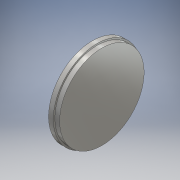
# Autodesk Inventor part: snow_can_top
Saved by Autodesk Inventor 2016 (Build 200138000, 138)
## iProperties
Created: 2017-01-14
Part Number: snow_can_top
Material: Generic
Document SubType Name: Modeling
Designer: hesaon
Density: 1 g/cm^3
Appearance: Default
Author: hesaon
Autodesk Inventor part; units mm, degrees
ref_plane "YZ Plane" through (0, 0, 0) normal (1, 0, 0) x (0, 1, 0)
ref_plane "XZ Plane" through (0, 0, 0) normal (0, 1, 0) x (-1, 0, 0)
ref_plane "XY Plane" through (0, 0, 0) normal (0, 0, 1) x (1, 0, 0)
sketch "Sketch1" plane through (0, 0, 0) normal (0, 1, 0) x (-1, 0, 0)
  line L0 (0, 27.75) -> (3, 27.75)
  line L1 (3, 27.75) -> (3, 25.75)
  line L2 (-3, 25.75) -> (-3, 23.75)
  line L3 (8, 13.5) -> (8, 0)
  line L4 (-3, 26.75) -> (-3, 0)
  line L5 (8, 0) -> (0, 0)
  arc A0 (8, 13.5) -> (0, 23.75) centre (-2.5664, 13.5) ccw
  arc A1 (0, 25.75) -> (0, 23.75) centre (0, 24.75) ccw
  line L6 (0, 26.75) -> (-3, 26.75)
  line L7 (-3, 26.75) -> (-3, 25.75)
  line L8 (3, 25.75) -> (0, 25.75)
  line L9 (0, 27.75) -> (0, 26.75)
  line L10 (0, 0) -> (-3, 0)
  line L11 (8, 0) -> (8, 16.2)
  line L12 (8, 16.2) -> (10.5, 16.2)
  line L13 (10.5, 16.2) -> (10.5, 14.7)
  line L14 (10.5, 14.7) -> (10.5, 13.7)
  line L15 (10.5, 13.7) -> (10.5, 12.2)
  line L16 (10.5, 12.2) -> (8, 12.2)
  line L17 (10.5, 14.7) -> (12, 14.7)
  line L18 (12, 14.7) -> (12, 13.7)
  line L19 (12, 13.7) -> (10.5, 13.7)
  arc A2 (12, 14.7) -> (10.5, 16.2) centre (10.5, 14.7) ccw
  arc A3 (10.5, 12.2) -> (12, 13.7) centre (10.5, 13.7) ccw
  dimension "d0" = 27.75
  dimension "d7" = 13.5
  dimension "d8" = 11
  dimension "d9" = 10.5664
  dimension "d10" = 1
  dimension "d11" = 3
  dimension "d12" = 3
  dimension "d14" = 16.2
  dimension "d15" = 2.5
  dimension "d16" = 1.5
  dimension "d17" = 1
  dimension "d18" = 1.5
  dimension "d19" = 1.5
  constraints: 40 end point, 8 perpendicular, 8 point on circle, 4 centre point, 4 horizontal, 4 point on line, 4 tangent, 4 vertical
  measures "d0" distance of L5.end L0.start
  measures "d7" distance of L3.end L3.start
  measures "d8" distance of L4.end L3.end
  measures "d9" radius of A0
  measures "d10" radius of A1
  measures "d11" distance of L4.start L6.start
  measures "d12" distance of L0.end L0.start
  measures "d14" distance of L3.end L11.end
  measures "d15" distance of L11.end L12.end
  measures "d16" distance of L12.end L13.end
  measures "d17" distance of L13.end L14.end
  measures "d18" distance of L14.end L15.end
  measures "d19" distance of L13.end L17.end
revolve "Revolution2" add sketch "Sketch1" angle 360 about axis through (-8, 0, 0) along (1, 0, 0)
body "Solid2"
